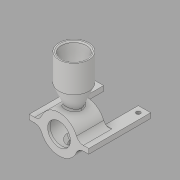
# Autodesk Inventor part: powderTurnRes
Saved by Autodesk Inventor 2017 (Build 210142000, 142)
## iProperties
Created: 2019-05-09
Part Number: powderTurnRes
Material: Generic
Document SubType Name: Modeling
Designer: Joe Sedutto
Density: 1 g/cm^3
Appearance: Default
Author: Joe Sedutto
Autodesk Inventor part; units mm, degrees
ref_plane "YZ Plane" through (0, 0, 0) normal (1, 0, 0) x (0, 1, 0)
ref_plane "XY Plane" through (0, 0, 0) normal (0, 0, 1) x (1, 0, 0)
sketch "Sketch1" plane through (0, 0, 0) normal (0, 0, 1) x (1, 0, 0)
  circle A0 centre (0, 0) radius 12.954
  circle A1 centre (0, 0) radius 19.304
  dimension "d0" = 25.908
  dimension "d1" = 6.35
  constraints: 2 centre point, 1 coincident
  measures "d0" diameter of A0
  measures "d1" radial gap between concentric circles of A0 A1
extrude "Extrusion1" add sketch "Sketch1" along normal blind 25.4
sketch "Sketch2" plane through (0, 0, 25.4) normal (0, 0, 1) x (1, 0, 0)
  circle A0 centre (0, 0) radius 12.954 projected
  circle A1 centre (0, 0) radius 19.304 projected
  circle A2 centre (0, 0) radius 11.684
  dimension "d4" = 1.27
  constraints: 1 centre point
  measures "d4" radial gap between concentric circles of A0 A2
extrude "Extrusion2" add sketch "Sketch2" along normal blind 2.54 contours A0 | A1
ref_plane "Work Plane1" through (0, 19.304, 0) normal (0, 1, 0) x (-1, 0, 0)
sketch "Sketch3" plane through (0, 19.304, 0) normal (0, 1, 0) x (-1, 0, 0)
  line L0 (-12.954, 0) -> (-12.954, 25.4) projected
  line L1 (0, 12.7) -> (-12.954, 12.7) construction
  line L2 (12.954, 0) -> (12.954, 25.4) projected
  line L3 (12.954, 12.7) -> (0, 12.7) construction
  point P0 (0, 0)
  constraints: 4 end point, 2 midpoint, 1 collinear, 1 horizontal
hole "Hole1" at (0, 19.304, 12.7) direction (0, -1, 0) diameter 6.35 depth 12.7 tip angle 118
ref_plane "Work Plane2" through (0, 0, 12.7) normal (0, 0, -1) x (-1, 0, 0)
sketch "Sketch4" plane through (0, 0, 12.7) normal (0, 0, -1) x (-1, 0, 0)
  line L0 (-3.175, 15.0989) -> (-12.7, 38.1)
  line L1 (-12.7, 38.1) -> (-15.24, 38.1)
  line L2 (-15.24, 38.1) -> (-5.715, 15.0989)
  line L3 (-5.715, 15.0989) -> (-3.175, 15.0989)
  circle A0 centre (0, 0) radius 19.304 projected
  line L4 (0, 19.304) -> (0, 32.8531) construction
  line L5 (-3.175, 12.5589) -> (-3.175, 19.0411) projected
  line L6 (0, 19.304) -> (0, 0) construction
  dimension "d15" = 2.54
  dimension "d16" = 38.1
  dimension "d18" = 2.54
  dimension "d51" = 15.24
  constraints: 12 end point, 2 parallel, 1 collinear, 1 horizontal, 1 point on circle, 1 point on line, 1 vertical
  measures "d15" distance of L0.end L1.end
  measures "d16" distance from line of L1 point (0, 0)
  measures "d18" distance of L0.start L5.start
  measures "d51" distance from line of L4 L1.end
revolve "Revolution1" add sketch "Sketch4" angle 360 about axis through (0, 19.304, 12.7) along (0, 1, 0) contours L3 L2 A0 L0 | A0 L2 L1 L0
sketch "Sketch5" plane through (0, 38.1, 12.7) normal (0, 1, 0) x (1, 0, 0)
  circle A0 centre (0, 0) radius 15.24 projected
  circle A1 centre (0, 0) radius 12.7 projected
  point P0 (0, 12.7)
extrude "Extrusion3" add sketch "Sketch5" along normal blind 27.94
fillet "Fillet1" radius 1.27 1 edges at (-12.7, 66.04, 12.7)
fillet "Fillet2" radius 1.27 1 edges at (-6.9244, 18.0194, 12.6991)
sketch "Sketch7" plane through (0, 0, 0) normal (0, 1, 0) x (-1, 0, 0)
  spline S0 degree 5 poles (0, 15.875) (0.3659, 15.875) (0.727, 15.8223) (1.0691, 15.7198) (1.3812, 15.5769) (2.0115, 15.1917) (2.3107, 14.9287) (2.5555, 14.637) (2.7488, 14.3277) (3.1275, 13.4884) (3.2362, 12.9392) (3.2299, 12.3841) (3.1079, 11.836) (2.6851, 10.958) (2.4465, 10.6104) (2.1388, 10.2882) (1.7587, 10.0103) (0.899, 9.6224) (0.426, 9.4951) (-0.0811, 9.4669) (-0.5725, 9.5429) (-1.4459, 9.8364) (-1.8265, 10.0515) (-2.1489, 10.3127) (-2.413, 10.6031) (-2.8481, 11.2412) (-3.0126, 11.5937) (-3.1209, 11.9587) (-3.175, 12.3291) (-3.175, 13.0562) (-3.1251, 13.4119) (-3.0253, 13.7628) (-2.8738, 14.1026) (-2.4642, 14.7368) (-2.2072, 15.0334) (-1.8917, 15.3023) (-1.5169, 15.5267) (-0.8852, 15.7566) (-0.6728, 15.8148) (-0.4518, 15.8549) (-0.2262, 15.875) (0, 15.875) knots 0 0 0 0 0 0 0.075675 0.075675 0.075675 0.075675 0.173848 0.173848 0.173848 0.173848 0.33165 0.33165 0.33165 0.33165 0.443629 0.443629 0.443629 0.443629 0.544215 0.544215 0.544215 0.544215 0.643873 0.643873 0.643873 0.643873 0.750434 0.750434 0.750434 0.750434 0.852758 0.852758 0.852758 0.852758 0.95322 0.95322 0.95322 0.95322 1 1 1 1 1 1
  spline S1 degree 5 poles (0, 17.145) (1.3934, 17.1441) (2.789, 16.6019) (3.8921, 15.4995) (4.9888, 12.716) (3.9097, 9.925) (2.8132, 8.8175) (0.0266, 7.709) (-2.7749, 8.7853) (-3.889, 9.8894) (-4.9936, 12.6867) (-3.9034, 15.488) (-2.7987, 16.5982) (-1.3982, 17.1441) (0, 17.145) knots 0 0 0 0 0 0 0.249517 0.249517 0.249517 0.498921 0.498921 0.498921 0.749622 0.749622 0.749622 1 1 1 1 1 1
  point P0 (0, 0)
  dimension "d30" = 1.27
  constraints: 3 other
extrude "Extrusion5" cut sketch "Sketch7" against normal blind 25.4 contours S0 | S1
chamfer "Chamfer2" distance 3.175 angle 45 1 edges at (0, -12.954, 8.2552)
sketch "Sketch8" plane through (0, 0, 0) normal (0, 1, 0) x (-1, 0, 0)
  line L0 (19.304, 27.94) -> (-19.304, 27.94) projected
  line L1 (17.78, 27.94) -> (30.48, 27.94)
  line L2 (30.48, 27.94) -> (30.48, -35.56)
  line L3 (30.48, -35.56) -> (17.78, -35.56)
  line L4 (17.78, -35.56) -> (17.78, 27.94)
  line L5 (0, 27.94) -> (0, -2.54) construction
  circle A0 centre (0, 12.7) radius 15.24 projected
  line L6 (-19.304, 27.94) -> (19.304, 27.94)
  line L7 (-17.78, 27.94) -> (-30.48, 27.94)
  line L8 (-30.48, 27.94) -> (-30.48, -35.56)
  line L9 (-30.48, -35.56) -> (-17.78, -35.56)
  line L10 (-17.78, -35.56) -> (-17.78, 27.94)
  circle A1 centre (0, 12.7) radius 15.24
  point P0 (0, 0)
  dimension "d36" = 12.7
  dimension "d37" = 17.78
  dimension "d38" = 63.5
  constraints: 20 end point, 6 symmetric about line, 2 parallel, 2 point on line, 1 centre point, 1 horizontal, 1 line through centre, 1 midpoint, 1 perpendicular, 1 vertical, 1 vertical alignment, 1 other
  measures "d36" distance between parallel lines of L4 L2
  measures "d37" distance from line of A1.centre L4
  measures "d38" distance between parallel lines of L1 L3
extrude "Extrusion6" add sketch "Sketch8" along normal mid plane 5.08 contours L1 L2 L3 L4 L0 | L10 L9 L8 L7 L0
fillet "Fillet3" radius 7.62 4 edges at (19.1362, 2.54, 13.97) (-19.1362, 2.54, 13.97) (-19.1362, -2.54, 13.97) (19.1362, -2.54, 13.97)
sketch "Sketch9" plane through (0, 2.54, 0) normal (0, 1, 0) x (1, 0, 0)
  line L0 (17.78, 35.56) -> (17.78, 0) projected
  line L1 (30.48, 35.56) -> (17.78, 35.56)
  line L2 (17.78, 35.56) -> (17.78, 22.86)
  line L3 (17.78, 22.86) -> (30.48, 22.86)
  line L4 (30.48, 22.86) -> (30.48, 35.56)
  line L5 (30.48, 35.56) -> (17.78, 22.86) construction
  line L6 (17.78, 35.56) -> (30.48, 22.86) construction
  line L7 (-30.48, -27.94) -> (-30.48, 35.56) projected
  line L8 (-17.78, 35.56) -> (-30.48, 35.56)
  line L9 (-30.48, 35.56) -> (-30.48, 22.86)
  line L10 (-30.48, 22.86) -> (-17.78, 22.86)
  line L11 (-17.78, 22.86) -> (-17.78, 35.56)
  line L12 (-17.78, 35.56) -> (-30.48, 22.86) construction
  line L13 (-30.48, 35.56) -> (-17.78, 22.86) construction
  line L14 (30.48, 35.56) -> (17.78, 35.56) projected
  line L15 (30.48, -27.94) -> (30.48, 35.56) projected
  line L16 (-17.78, 35.56) -> (-30.48, 35.56) projected
  line L17 (-17.78, 0) -> (-17.78, 35.56) projected
  point P0 (0, 0)
  point P1 (24.13, 29.21)
  point P2 (-24.13, 29.21)
  point P3 (24.13, 29.21)
  point P4 (-24.13, 29.21)
  constraints: 24 end point, 4 collinear, 4 midpoint, 4 parallel, 3 perpendicular, 3 point on line, 2 coincident, 2 horizontal
hole "Hole2" at (24.13, 2.54, -29.21) at (-24.13, 2.54, -29.21) direction (0, -1, 0) diameter 4.2333 depth 12.7 tip angle 118
fillet "Fillet4" radius 1.27 4 edges at (21.3567, 2.54, 0) (-21.3567, 2.54, 0) (-21.3567, -2.54, 0) (21.3567, -2.54, 0)
fillet "Fillet5" radius 1.27 6 edges at (-17.78, -3.175, 0) (-17.78, 0, 0) (-17.78, 3.175, 0) (17.78, -3.175, 0) (17.78, 0, 0) (17.78, 3.175, 0)
body "Solid1"
